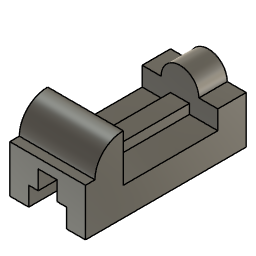
Task2Done v0 (Autodesk Fusion 360 design; units mm, degrees)
Autodesk Fusion 360 part; units mm, degrees
sketch "Sketch1" plane through (0, 0, 0) normal (0, 0, 1) x (1, 0, 0)
  line L0 (0, 0) -> (8, 0)
  line L1 (8, 0) -> (8, 17)
  line L2 (8, 17) -> (0, 17)
  line L3 (0, 17) -> (0, 0)
  dimension "d1" = 8
  dimension "d2" = 17
  constraint horizontal L0
  constraint vertical L1
  constraint horizontal L2
  constraint vertical L3
  constraint coincident L0.start L3.end
  measures "d1" distance of L0.start L0.end
  measures "d2" distance of L0.start L2.end
extrude "Extrude1" add sketch "Sketch1" along normal blind 3
sketch "Sketch2" plane through (0, 0, 3) normal (0, 0, 1) x (-1, 0, 0)
  line L0 (0, -17) -> (0, 0)
  line L1 (0, 0) -> (-8, 0)
  line L2 (-8, 0) -> (-8, -17)
  line L3 (-8, -17) -> (0, -17)
  line L4 (0, 0) -> (-8, 0)
  line L5 (-8, 0) -> (-8, -4)
  line L6 (-8, -4) -> (0, -4)
  line L7 (0, -4) -> (0, 0)
  dimension "d5" = 8
  dimension "d6" = 4
  constraint horizontal L4
  constraint vertical L5
  constraint horizontal L6
  constraint vertical L7
  constraint coincident L0.end L1.start
  measures "d5" distance of L0.end L1.end
  measures "d6" distance of L0.end L6.end
extrude "Extrude2" add sketch "Sketch2" along normal blind 2 contours L0 L1 L2 L4 L5 L6 L7
sketch "Sketch3" plane through (0, 0, 5) normal (0, 0, 1) x (-1, 0, 0)
  line L0 (0, -4) -> (0, 0)
  line L1 (0, 0) -> (-8, 0)
  line L2 (-8, 0) -> (-8, -4)
  line L3 (-8, -4) -> (0, -4)
  line L4 (0, 0) -> (-8, 0)
  line L5 (-8, 0) -> (-8, -1)
  line L6 (-8, -1) -> (0, -1)
  line L7 (0, -1) -> (0, 0)
  dimension "d9" = 8
  constraint horizontal L4
  constraint vertical L5
  constraint horizontal L6
  constraint vertical L7
  constraint coincident L0.end L1.start
  measures "d9" distance of L0.end L1.end
extrude "Extrude3" add sketch "Sketch3" along normal blind 3 contours L0 L2 L3 L6
fillet "Fillet1" radius 3 1 edges at (4, 1, 8)
sketch "Sketch4" plane through (0, 0, 3) normal (0, 0, 1) x (-1, 0, 0)
  line L0 (0, -4) -> (-8, -4)
  line L1 (-8, -4) -> (-8, -17)
  line L2 (-8, -17) -> (0, -17)
  line L3 (0, -17) -> (0, -4)
  line L4 (0, -17) -> (-8, -17)
  line L5 (-8, -17) -> (-8, -14)
  line L6 (-8, -14) -> (0, -14)
  line L7 (0, -14) -> (0, -17)
  dimension "d14" = 3
  constraint horizontal L4
  constraint vertical L5
  constraint horizontal L6
  constraint vertical L7
  constraint coincident L2.end L3.start
  measures "d14" distance of L2.end L6.end
extrude "Extrude4" add sketch "Sketch4" along normal blind 2 contours L1 L2 L3 L4 L5 L6 L7
sketch "Sketch5" plane through (0, 0, 5) normal (0, 0, 1) x (-1, 0, 0)
  line L0 (0, -14) -> (-8, -14)
  line L1 (-8, -14) -> (-8, -17)
  line L2 (-8, -17) -> (0, -17)
  line L3 (0, -17) -> (0, -14)
  line L4 (-8, -17) -> (-6, -17)
  line L5 (-6, -17) -> (-6, -14)
  line L6 (-6, -14) -> (-8, -14)
  line L7 (-8, -14) -> (-8, -17)
  line L8 (0, -17) -> (-2, -17)
  line L9 (-2, -17) -> (-2, -14)
  line L10 (-2, -14) -> (0, -14)
  line L11 (0, -14) -> (0, -17)
  dimension "d17" = 2
  dimension "d18" = 2
  constraint horizontal L4
  constraint vertical L5
  constraint horizontal L6
  constraint vertical L7
  constraint coincident L1.end L2.start
  constraint horizontal L8
  constraint vertical L9
  constraint horizontal L10
  constraint vertical L11
  constraint coincident L2.end L3.start
  measures "d17" distance of L1.end L4.end
  measures "d18" distance of L2.end L8.end
extrude "Extrude5" add sketch "Sketch5" along normal blind 2 contours L0 L2 L5 L9
fillet "Fillet2" radius 2 2 edges at (2, 15.5, 7) (6, 15.5, 7)
sketch "Sketch6" plane through (0, 0, 0) normal (0, -1, 0) x (1, 0, 0)
  line L0 (0, 0) -> (8, 0)
  line L1 (8, 0) -> (8, 5)
  line L2 (8, 5) -> (0, 5)
  line L3 (0, 5) -> (0, 0)
  line L4 (0, 0) -> (2, 0)
  line L5 (2, 0) -> (2, 2)
  line L6 (2, 2) -> (0, 2)
  line L7 (0, 2) -> (0, 0)
  line L8 (8, 0) -> (6, 0)
  line L9 (6, 0) -> (6, 2)
  line L10 (6, 2) -> (8, 2)
  line L11 (8, 2) -> (8, 0)
  line L12 (2, 2) -> (6, 2)
  line L13 (6, 2) -> (6, 0)
  line L14 (6, 0) -> (2, 0)
  line L15 (2, 0) -> (2, 2)
  dimension "d23" = 2
  dimension "d24" = 2
  dimension "d25" = 2
  constraint horizontal L4
  constraint vertical L5
  constraint horizontal L6
  constraint vertical L7
  constraint coincident L0.start L3.end
  constraint horizontal L8
  constraint vertical L9
  constraint horizontal L10
  constraint vertical L11
  constraint coincident L0.end L1.start
  constraint horizontal L12
  constraint vertical L13
  constraint horizontal L14
  constraint vertical L15
  measures "d23" distance of L0.start L4.end
  measures "d24" distance of L0.start L6.end
  measures "d25" distance of L0.end L8.end
extrude "Extrude6" cut sketch "Sketch6" against normal blind 23 contours L0 L5 L9 L12 L13 L14 L15
sketch "Sketch7" plane through (0, 0, 3) normal (0, 0, 1) x (-1, 0, 0)
  line L0 (-8, -14) -> (0, -14)
  line L1 (0, -14) -> (0, -4)
  line L2 (0, -4) -> (-8, -4)
  line L3 (-8, -4) -> (-8, -14)
  line L4 (0, -4) -> (-3, -4)
  line L5 (-3, -4) -> (-3, -14)
  line L6 (-3, -14) -> (0, -14)
  line L7 (0, -14) -> (0, -4)
  line L8 (-8, -4) -> (-5, -4)
  line L9 (-5, -4) -> (-5, -14)
  line L10 (-5, -14) -> (-8, -14)
  line L11 (-8, -14) -> (-8, -4)
  dimension "d28" = 3
  dimension "d29" = 3
  constraint horizontal L4
  constraint vertical L5
  constraint horizontal L6
  constraint vertical L7
  constraint coincident L1.end L2.start
  constraint horizontal L8
  constraint vertical L9
  constraint horizontal L10
  constraint vertical L11
  constraint coincident L2.end L3.start
  measures "d28" distance of L1.end L4.end
  measures "d29" distance of L2.end L8.end
extrude "Extrude7" add sketch "Sketch7" along normal blind 1 contours L0 L2 L5 L9
sketch "Sketch8" plane through (0, 0, 2) normal (0, 0, -1) x (1, 0, 0)
  line L0 (2, -17) -> (6, -17)
  line L1 (6, -17) -> (6, 0)
  line L2 (6, 0) -> (2, 0)
  line L3 (2, 0) -> (2, -17)
  line L4 (6, 0) -> (2, 0)
  line L5 (2, 0) -> (2, -4)
  line L6 (2, -4) -> (6, -4)
  line L7 (6, -4) -> (6, 0)
  line L8 (6, 0) -> (5, 0)
  line L9 (5, 0) -> (5, -4)
  line L10 (5, -4) -> (6, -4)
  line L11 (6, -4) -> (6, 0)
  line L12 (2, 0) -> (3, 0)
  line L13 (3, 0) -> (3, -4)
  line L14 (3, -4) -> (2, -4)
  line L15 (2, -4) -> (2, 0)
  line L16 (6, -17) -> (2, -17)
  line L17 (2, -17) -> (2, -14)
  line L18 (2, -14) -> (6, -14)
  line L19 (6, -14) -> (6, -17)
  line L20 (6, -17) -> (5, -17)
  line L21 (5, -17) -> (5, -14)
  line L22 (5, -14) -> (6, -14)
  line L23 (6, -14) -> (6, -17)
  line L24 (2, -17) -> (3, -17)
  line L25 (3, -17) -> (3, -14)
  line L26 (3, -14) -> (2, -14)
  line L27 (2, -14) -> (2, -17)
  dimension "d32" = 4
  dimension "d33" = 1
  dimension "d34" = 1
  dimension "d35" = 3
  dimension "d36" = 1
  dimension "d37" = 1
  constraint horizontal L4
  constraint vertical L5
  constraint horizontal L6
  constraint vertical L7
  constraint coincident L1.end L2.start
  constraint horizontal L8
  constraint vertical L9
  constraint horizontal L10
  constraint vertical L11
  constraint horizontal L12
  constraint vertical L13
  constraint horizontal L14
  constraint vertical L15
  constraint horizontal L16
  constraint vertical L17
  constraint horizontal L18
  constraint vertical L19
  constraint coincident L0.end L1.start
  constraint horizontal L20
  constraint vertical L21
  constraint horizontal L22
  constraint vertical L23
  constraint horizontal L24
  constraint vertical L25
  constraint horizontal L26
  constraint vertical L27
  measures "d32" distance of L1.end L6.end
  measures "d33" distance of L1.end L8.end
  measures "d34" distance of L2.end L12.end
  measures "d35" distance of L0.end L18.end
  measures "d36" distance of L0.end L20.end
  measures "d37" distance of L0.start L24.end
extrude "Extrude8" cut sketch "Sketch8" against normal blind 2 contours L0 L16 L18 L21 L25 | L2 L4 L6 L9 L13
